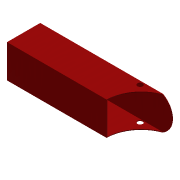
# Autodesk Inventor part: Case
Saved by Autodesk Inventor 2015 (Build 190159000, 159)
## iProperties
Created: 2015-01-07
Part Number: Case
Material: Všeobecné
Document SubType Name: Modeling
Designer: Michal
Density: 1 g/cm^3
Appearance: Červená
Author: Michal
Autodesk Inventor part; units mm, degrees
ref_plane "YZ Plane" through (0, 0, 0) normal (1, 0, 0) x (0, 1, 0)
ref_plane "XZ Plane" through (0, 0, 0) normal (0, 1, 0) x (-1, 0, 0)
ref_plane "XY Plane" through (0, 0, 0) normal (0, 0, 1) x (1, 0, 0)
sketch "Náčrt1" plane through (0, 0, 0) normal (1, 0, 0) x (0, 1, 0)
  line L0 (0, 0) -> (100, 0)
  line L1 (100, 0) -> (100, -100)
  line L2 (100, -100) -> (0, -100)
  line L3 (0, -100) -> (0, 0)
  line L4 (98, -2) -> (2, -2)
  line L5 (2, -2) -> (2, -98)
  line L6 (2, -98) -> (98, -98)
  line L7 (98, -98) -> (98, -2)
  dimension "d0" = 100
  dimension "d1" = 100
  dimension "d2" = 2
  constraints: 16 end point, 4 parallel, 2 perpendicular, 1 horizontal, 3 other
  measures "d0" distance of L1.end L2.end
  measures "d1" distance of L0.end L1.end
  measures "d2" distance between parallel lines of L0 L4
extrude "Vysunutí1" add sketch "Náčrt1" along normal blind 370
sketch "Náčrt4" plane through (0, 0, 0) normal (0, 0, 1) x (1, 0, 0)
  circle A0 centre (406.7759, -2.2685) radius 106.8
  line L0 (0, 0) -> (0, 100) projected
  line L1 (0, 0) -> (370, 0) projected
  line L2 (370, 100) -> (370, 0) projected
  line L3 (0, 100) -> (370, 100) projected
  line L4 (300, 0) -> (370, 0)
  line L5 (370, 0) -> (370, 98)
  dimension "d16" = 213.6
  dimension "d17" = 2
  dimension "d18" = 300
  constraints: 4 end point, 2 point on circle, 2 point on line, 1 centre point, 1 collinear, 1 horizontal
  measures "d16" diameter of A0
  measures "d17" distance from line of L3 L5.end
  measures "d18" distance of point (0, 0) L4.start
extrude "Vysunutí4" cut sketch "Náčrt4" against normal through all contours L2 L1 A0 picked at (365.6726, 63.4107)
sketch "Náčrt5" plane through (0, 100, 0) normal (0, 1, 0) x (1, 0, 0)
  line L0 (0, 0) -> (0, 100) projected
  line L1 (0, 0) -> (370, 0) projected
  line L2 (370, 100) -> (370, 0) projected
  line L3 (0, 100) -> (370, 100) projected
  arc A0 (370, 0) -> (370, 100) centre (343.3333, 50) ccw
  point P0 (400, 50)
  dimension "d21" = 30
  constraints: 3 point on circle, 1 centre point
  measures "d21" distance from line of point (400, 50) L2
extrude "Vysunutí5" add sketch "Náčrt5" against normal blind 2 contours L2 A0
sketch "Náčrt6" plane through (0, 0, 0) normal (0, 0, 1) x (1, 0, 0)
  arc A0 (370, 98) -> (300, 0) centre (406.7759, -2.2685) ccw projected
  line L0 (370, 100) -> (370, 98) projected
  line L1 (0, 100) -> (370, 100) projected
  line L2 (0, 0) -> (0, 100) projected
  line L3 (0, 0) -> (300, 0) projected
  circle A1 centre (312, 89) radius 8
  dimension "d24" = 16
  dimension "d25" = 11
  dimension "d26" = 312
  constraints: 1 centre point
  measures "d24" diameter of A1
  measures "d25" distance from line of L1 A1.centre
  measures "d26" distance from line of L2 A1.centre
extrude "Vysunutí6" cut sketch "Náčrt6" against normal through all contours A1
